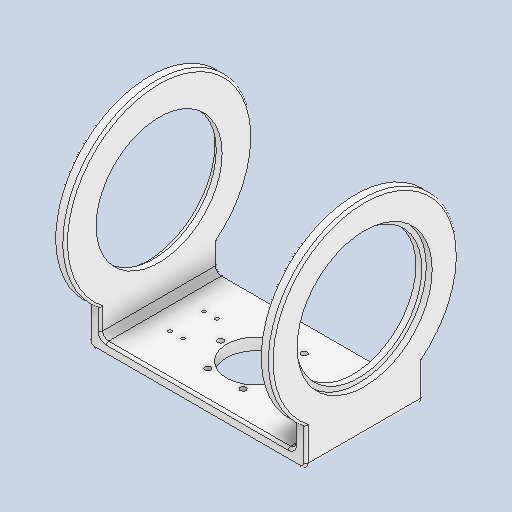
# Autodesk Inventor part: base
Saved by Autodesk Inventor 2025.3 (Build 293356030, 356C)
## iProperties
Created: 2025-08-30
Part Number: base
Material: PLA+ filament
Document SubType Name: Modeling
Designer: MSI
Density: 1.23 g/cm^3
Appearance: 일반
Mass: 480.42 g
Surface Area: 1009.74 cm^2
Volume: 390.586 cm^3
Author: MSI
Autodesk Inventor part; units mm, degrees
ref_plane "YZ Plane" through (0, 0, 0) normal (1, 0, 0) x (0, 1, 0)
ref_plane "XZ Plane" through (0, 0, 0) normal (0, 1, 0) x (-1, 0, 0)
ref_plane "XY Plane" through (0, 0, 0) normal (0, 0, 1) x (1, 0, 0)
sketch "스케치1" plane through (0, 0, 0) normal (1, 0, 0) x (0, 1, 0)
  circle A0 centre (0, 0) radius 80
  line L0 (0, 50) -> (-95, 50)
  line L1 (-95, 50) -> (-95, -50)
  line L2 (-95, -50) -> (0, -50)
  line L3 (0, -50) -> (0, 50)
  point P0 (-95, 0)
  point P1 (-62.45, -50)
  point P2 (-62.45, 50)
  dimension "d0" = 160
  dimension "d1" = 95
  dimension "d36" = 100
  constraints: 8 end point, 2 coincident, 2 midpoint, 2 parallel, 1 centre point, 1 horizontal, 1 horizontal alignment, 1 perpendicular
  measures "d0" diameter of A0
  measures "d1" distance of L1.end L2.end
  measures "d36" distance of L0.end L1.end
extrude "돌출1" add sketch "스케치1" along normal mid plane 185
sketch "스케치2" plane through (0, 0, 0) normal (0, 0, 1) x (1, 0, 0)
  line L0 (-92.5, 80) -> (92.5, 80) projected
  line L1 (-82.5, 80) -> (82.5, 80)
  line L2 (82.5, 80) -> (82.5, -85)
  line L3 (82.5, -85) -> (-82.5, -85)
  line L4 (-82.5, -85) -> (-82.5, 80)
  line L5 (-92.5, -95) -> (92.5, -95) projected
  line L6 (92.5, -95) -> (92.5, -62.45) projected
  point P0 (0, 0)
  point P1 (0, -85)
  dimension "d4" = 10
  dimension "d5" = 10
  constraints: 8 end point, 2 parallel, 1 horizontal, 1 midpoint, 1 perpendicular, 1 point on line, 1 vertical alignment
  measures "d4" distance between parallel lines of L5 L3
  measures "d5" distance between parallel lines of L6 L2
extrude "돌출2" cut sketch "스케치2" along normal through all both and the other way through all
sketch "스케치3" plane through (-82.5, -85, -50) normal (0, 1, 0) x (1, 0, 0)
  point P0 (82.5, -50)
  point P1 (82.5, -50)
  constraints: 1 coincident
hole "구멍1" at (0, -85, 0) direction (0, -1, 0) diameter 50 end through all
sketch "스케치4" plane through (92.5, 0, 0) normal (1, 0, 0) x (0, 0, -1)
  arc A0 (50, -62.45) -> (-50, -62.45) centre (0, 0) ccw projected
  point P0 (-80, 0)
  constraints: 1 coincident
hole "구멍2" at (92.5, 0, 0) direction (-1, 0, 0) diameter 107.25 end through all counterbore diameter 115 counterbore depth 5
mirror "미러1" about plane through (0, 0, 0) normal (1, 0, 0) of "구멍2"
fillet "모깎기1" radius 5 2 edges at (-82.5, -85, 0) (82.5, -85, 0)
fillet "모깎기2" radius 5 2 edges at (92.5, -95, 0) (-92.5, -95, 0)
fillet "모깎기3" radius 2 24 edges at (-82.5, 80, 0) (-82.5, -71.225, -50) (-81.0355, -83.5355, -50) (0, -85, -50) (81.0355, -83.5355, -50) (82.5, -71.225, -50) (82.5, 80, 0) (82.5, -71.225, 50) (81.0355, -83.5355, 50) (0, -85, 50) (-81.0355, -83.5355, 50) (-82.5, -71.225, 50) (-92.5, 80, 0) (-92.5, -76.225, -50) (-91.0355, -93.5355, -50) (0, -95, -50) (91.0355, -93.5355, -50) (92.5, -76.225, -50) (92.5, 80, 0) (92.5, -76.225, 50) (91.0355, -93.5355, 50) (0, -95, 50) (-91.0355, -93.5355, 50) (-92.5, -76.225, 50)
sketch "스케치5" plane through (-77.5, -85, -48) normal (0, 1, 0) x (1, 0, 0)
  line L0 (77.5, -48) -> (47.5, -48) construction
  dimension "d25" = 30
  constraints: 2 end point, 1 horizontal
  measures "d25" distance of L0.start L0.end
hole "구멍3" at (-30, -85, 0) direction (0, -1, 0) diameter 5 end through all
pattern_circular "원형 패턴1" count 6 over 360 about axis through (0, -385.7491, 0) along (0, 1, 0) of "구멍3"
sketch "스케치6" plane through (-77.5, -85, -48) normal (0, 1, 0) x (1, 0, 0)
  line L0 (16.721, -31.5) -> (31.721, -31.5)
  line L1 (31.721, -31.5) -> (31.721, -64.5)
  line L2 (31.721, -64.5) -> (16.721, -64.5)
  line L3 (16.721, -64.5) -> (16.721, -31.5)
  line L4 (16.721, -31.5) -> (31.721, -64.5) construction
  line L5 (31.721, -31.5) -> (16.721, -64.5) construction
  circle A0 centre (77.5, -48) radius 25 projected
  line L6 (77.5, -23) -> (77.5, -73) construction
  line L7 (138.279, -31.5) -> (123.279, -31.5)
  line L8 (123.279, -31.5) -> (123.279, -64.5)
  line L9 (123.279, -64.5) -> (138.279, -64.5)
  line L10 (138.279, -64.5) -> (138.279, -31.5)
  line L11 (138.279, -31.5) -> (123.279, -64.5) construction
  line L12 (123.279, -31.5) -> (138.279, -64.5) construction
  line L13 (29.721, -62.5) -> (29.721, -33.5)
  line L14 (29.721, -33.5) -> (18.721, -33.5)
  line L15 (18.721, -33.5) -> (18.721, -62.5)
  line L16 (18.721, -62.5) -> (29.721, -62.5)
  line L17 (136.279, -62.5) -> (125.279, -62.5)
  line L18 (125.279, -62.5) -> (125.279, -33.5)
  line L19 (125.279, -33.5) -> (136.279, -33.5)
  line L20 (136.279, -33.5) -> (136.279, -62.5)
  point P0 (24.221, -48)
  point P1 (130.779, -48)
  dimension "d37" = 45.779
  dimension "d38" = 15
  dimension "d39" = 33
  dimension "d47" = 2
  dimension "d48" = 2
  constraints: 42 end point, 5 symmetric about line, 4 parallel, 3 midpoint, 2 perpendicular, 2 point on circle, 1 coincident, 1 horizontal, 1 horizontal alignment, 1 vertical, 6 other
  measures "d37" distance from line of point (77.5, -48) L1
  measures "d38" distance of L1.end L2.end
  measures "d39" distance of L2.end L0.start
  measures "d47" distance between parallel lines of L1 L13
  measures "d48" distance between parallel lines of L9 L17
hole "구멍4" at (47.779, -85, 14.5) at (47.779, -85, -14.5) at (58.779, -85, -14.5) at (58.779, -85, 14.5) at (-47.779, -85, -14.5) at (-47.779, -85, 14.5) at (-58.779, -85, 14.5) at (-58.779, -85, -14.5) direction (0, -1, 0) diameter 2.9 end through all clearance for "Flat Head Machine Screw" size "M2.5" standard "Ansi Metric M Profile"
equation "\"d5\" = d4"
